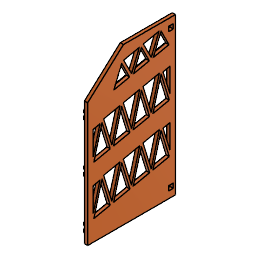
side-panel-right (Autodesk Fusion 360 design; units mm, degrees)
part number: 2026-08-18-20-37-21-779
Autodesk Fusion 360 part; units mm, degrees
sketch "Sketch1" plane through (0, 0, 0) normal (1, 0, 0) x (0, 0, -1)
  line L0 (0, 15) -> (0, 150)
  line L1 (0, 150) -> (-240, 150)
  line L2 (-240, 150) -> (-240, 70)
  line L3 (-240, 70) -> (-190, 15)
  line L4 (-190, 15) -> (0, 15)
extrude "Extrude1" add sketch "Sketch1" along normal blind 5 from surface at 6 makes body 1
sketch "Sketch2" plane through (0, 0, 0) normal (1, 0, 0) x (0, 0, -1)
  line L0 (-9, 20) -> (-35.5696, 145)
  line L1 (-35.5696, 145) -> (-41.5696, 145)
  line L2 (-41.5696, 145) -> (-15, 20)
  line L3 (-15, 20) -> (-9, 20)
extrude "Extrude2" add sketch "Sketch2" along normal blind 6 separate body makes body 2
sketch "Sketch3" plane through (0, 0, 0) normal (1, 0, 0) x (0, 0, -1)
  line L0 (-18.2, 20) -> (-44.7696, 145)
  line L1 (-44.7696, 145) -> (-49.7696, 145)
  line L2 (-49.7696, 145) -> (-23.2, 20)
  line L3 (-23.2, 20) -> (-18.2, 20)
extrude "Extrude3" add sketch "Sketch3" along normal blind 6 separate body makes body 3
sketch "Sketch4" plane through (0, 0, 0) normal (1, 0, 0) x (0, 0, -1)
  line L0 (-16.2753, 26) -> (-17.2753, 28)
  line L1 (-17.2753, 28) -> (-18.3381, 31)
  line L2 (-18.3381, 31) -> (-17.7632, 33)
  line L3 (-17.7632, 33) -> (-16.2753, 26)
extrude "Extrude4" add sketch "Sketch4" along normal blind 6 separate body makes body 4
sketch "Sketch5" plane through (0, 0, 0) normal (1, 0, 0) x (0, 0, -1)
  line L0 (-84, 20) -> (-110.5696, 145)
  line L1 (-110.5696, 145) -> (-116.5696, 145)
  line L2 (-116.5696, 145) -> (-90, 20)
  line L3 (-90, 20) -> (-84, 20)
extrude "Extrude5" add sketch "Sketch5" along normal blind 6 separate body makes body 5
sketch "Sketch6" plane through (0, 0, 0) normal (1, 0, 0) x (0, 0, -1)
  line L0 (-93.2, 20) -> (-119.7696, 145)
  line L1 (-119.7696, 145) -> (-124.7696, 145)
  line L2 (-124.7696, 145) -> (-98.2, 20)
  line L3 (-98.2, 20) -> (-93.2, 20)
extrude "Extrude6" add sketch "Sketch6" along normal blind 6 separate body makes body 6
sketch "Sketch7" plane through (0, 0, 0) normal (1, 0, 0) x (0, 0, -1)
  line L0 (-91.2753, 26) -> (-92.2753, 28)
  line L1 (-92.2753, 28) -> (-93.3381, 31)
  line L2 (-93.3381, 31) -> (-92.7632, 33)
  line L3 (-92.7632, 33) -> (-91.2753, 26)
extrude "Extrude7" add sketch "Sketch7" along normal blind 6 separate body makes body 7
sketch "Sketch8" plane through (0, 0, 0) normal (1, 0, 0) x (0, 0, -1)
  line L0 (-159, 20) -> (-185.5696, 145)
  line L1 (-185.5696, 145) -> (-191.5696, 145)
  line L2 (-191.5696, 145) -> (-165, 20)
  line L3 (-165, 20) -> (-159, 20)
extrude "Extrude8" add sketch "Sketch8" along normal blind 6 separate body makes body 8
sketch "Sketch9" plane through (0, 0, 0) normal (1, 0, 0) x (0, 0, -1)
  line L0 (-168.2, 20) -> (-194.7696, 145)
  line L1 (-194.7696, 145) -> (-199.7696, 145)
  line L2 (-199.7696, 145) -> (-173.2, 20)
  line L3 (-173.2, 20) -> (-168.2, 20)
extrude "Extrude9" add sketch "Sketch9" along normal blind 6 separate body makes body 9
sketch "Sketch10" plane through (0, 0, 0) normal (1, 0, 0) x (0, 0, -1)
  line L0 (-166.2753, 26) -> (-167.2753, 28)
  line L1 (-167.2753, 28) -> (-168.3381, 31)
  line L2 (-168.3381, 31) -> (-167.7632, 33)
  line L3 (-167.7632, 33) -> (-166.2753, 26)
extrude "Extrude10" add sketch "Sketch10" along normal blind 6 separate body makes body 10
combine "Combine1" operation add target body 1 tool bodies 2 3 4 5 6 7 8 9 10
sketch "Sketch11" plane through (0, 0, 0) normal (1, 0, 0) x (0, 0, -1)
  line L0 (-10.5, 139.5) -> (-10.5, 146.5)
  line L1 (-10.5, 146.5) -> (-17.5, 146.5)
  line L2 (-17.5, 146.5) -> (-17.5, 139.5)
  line L3 (-17.5, 139.5) -> (-10.5, 139.5)
extrude "Extrude11" cut sketch "Sketch11" along normal blind 30 from surface at -2 bodies 1
sketch "Sketch12" plane through (0, 0, 0) normal (1, 0, 0) x (0, 0, -1)
  line L0 (-222.5, 139.5) -> (-222.5, 146.5)
  line L1 (-222.5, 146.5) -> (-229.5, 146.5)
  line L2 (-229.5, 146.5) -> (-229.5, 139.5)
  line L3 (-229.5, 139.5) -> (-222.5, 139.5)
extrude "Extrude12" cut sketch "Sketch12" along normal blind 30 from surface at -2 bodies 1
sketch "Sketch13" plane through (0, 0, 0) normal (1, 0, 0) x (0, 0, -1)
  line L0 (-31.2766, 24.6534) -> (-36.5785, 49.5966)
  line L1 (-36.5785, 49.5966) -> (-77.4649, 37.125)
  line L2 (-77.4649, 37.125) -> (-31.2766, 24.6534)
  line L3 (-37.7065, 54.9034) -> (-43.0083, 79.8466)
  line L4 (-43.0083, 79.8466) -> (-83.8948, 67.375)
  line L5 (-83.8948, 67.375) -> (-37.7065, 54.9034)
  line L6 (-44.1363, 85.1534) -> (-49.4382, 110.0966)
  line L7 (-49.4382, 110.0966) -> (-90.3246, 97.625)
  line L8 (-90.3246, 97.625) -> (-44.1363, 85.1534)
  line L9 (-50.5662, 115.4034) -> (-55.868, 140.3466)
  line L10 (-55.868, 140.3466) -> (-96.7545, 127.875)
  line L11 (-96.7545, 127.875) -> (-50.5662, 115.4034)
  line L12 (-81.1165, 39.7784) -> (-86.4183, 64.7216)
  line L13 (-86.4183, 64.7216) -> (-40.23, 52.25)
  line L14 (-40.23, 52.25) -> (-81.1165, 39.7784)
  line L15 (-87.5463, 70.0284) -> (-92.8482, 94.9716)
  line L16 (-92.8482, 94.9716) -> (-46.6599, 82.5)
  line L17 (-46.6599, 82.5) -> (-87.5463, 70.0284)
  line L18 (-93.9761, 100.2784) -> (-99.278, 125.2216)
  line L19 (-99.278, 125.2216) -> (-53.0897, 112.75)
  line L20 (-53.0897, 112.75) -> (-93.9761, 100.2784)
  line L21 (-38.7844, 23.5511) -> (-75.34, 23.5511)
  line L22 (-75.34, 23.5511) -> (-77.5658, 34.0228)
  line L23 (-77.5658, 34.0228) -> (-38.7844, 23.5511)
  line L24 (-63.8444, 141.4489) -> (-100.3999, 141.4489)
  line L25 (-100.3999, 141.4489) -> (-98.1741, 130.9772)
  line L26 (-98.1741, 130.9772) -> (-63.8444, 141.4489)
  line L27 (-106.2766, 24.6534) -> (-111.5785, 49.5966)
  line L28 (-111.5785, 49.5966) -> (-152.4649, 37.125)
  line L29 (-152.4649, 37.125) -> (-106.2766, 24.6534)
  line L30 (-112.7065, 54.9034) -> (-118.0083, 79.8466)
  line L31 (-118.0083, 79.8466) -> (-158.8948, 67.375)
  line L32 (-158.8948, 67.375) -> (-112.7065, 54.9034)
  line L33 (-119.1363, 85.1534) -> (-124.4382, 110.0966)
  line L34 (-124.4382, 110.0966) -> (-165.3246, 97.625)
  line L35 (-165.3246, 97.625) -> (-119.1363, 85.1534)
  line L36 (-125.5662, 115.4034) -> (-130.868, 140.3466)
  line L37 (-130.868, 140.3466) -> (-171.7545, 127.875)
  line L38 (-171.7545, 127.875) -> (-125.5662, 115.4034)
  line L39 (-156.1165, 39.7784) -> (-161.4183, 64.7216)
  line L40 (-161.4183, 64.7216) -> (-115.23, 52.25)
  line L41 (-115.23, 52.25) -> (-156.1165, 39.7784)
  line L42 (-162.5463, 70.0284) -> (-167.8482, 94.9716)
  line L43 (-167.8482, 94.9716) -> (-121.6599, 82.5)
  line L44 (-121.6599, 82.5) -> (-162.5463, 70.0284)
  line L45 (-168.9761, 100.2784) -> (-174.278, 125.2216)
  line L46 (-174.278, 125.2216) -> (-128.0897, 112.75)
  line L47 (-128.0897, 112.75) -> (-168.9761, 100.2784)
  line L48 (-113.7844, 23.5511) -> (-150.34, 23.5511)
  line L49 (-150.34, 23.5511) -> (-152.5658, 34.0228)
  line L50 (-152.5658, 34.0228) -> (-113.7844, 23.5511)
  line L51 (-138.8444, 141.4489) -> (-175.3999, 141.4489)
  line L52 (-175.3999, 141.4489) -> (-173.1741, 130.9772)
  line L53 (-173.1741, 130.9772) -> (-138.8444, 141.4489)
  line L54 (-186.9937, 55.355) -> (-192.1035, 79.395)
  line L55 (-192.1035, 79.395) -> (-216.0124, 67.375)
  line L56 (-216.0124, 67.375) -> (-186.9937, 55.355)
  line L57 (-193.4235, 85.605) -> (-198.5334, 109.645)
  line L58 (-198.5334, 109.645) -> (-222.4422, 97.625)
  line L59 (-222.4422, 97.625) -> (-193.4235, 85.605)
  line L60 (-199.8534, 115.855) -> (-204.9632, 139.895)
  line L61 (-204.9632, 139.895) -> (-228.8721, 127.875)
  line L62 (-228.8721, 127.875) -> (-199.8534, 115.855)
  line L63 (-218.9511, 70.48) -> (-224.061, 94.52)
  line L64 (-224.061, 94.52) -> (-195.0423, 82.5)
  line L65 (-195.0423, 82.5) -> (-218.9511, 70.48)
  line L66 (-225.381, 100.73) -> (-230.4908, 124.77)
  line L67 (-230.4908, 124.77) -> (-201.4721, 112.75)
  line L68 (-201.4721, 112.75) -> (-225.381, 100.73)
extrude "Extrude13" cut sketch "Sketch13" along normal blind 9 from surface at 4 bodies 1
named bodies: "Тело"
